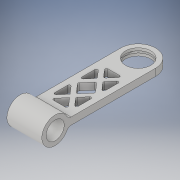
# Autodesk Inventor part: motor test flapper
Saved by Autodesk Inventor 2018.2 (Build 222227000, 227)
## iProperties
Created: 2018-03-04
Part Number: motor test flapper
Material: Generic
Document SubType Name: Modeling
Designer: torba
Density: 1 g/cm^3
Appearance: Default
Author: torba
Autodesk Inventor part; units mm, degrees
ref_plane "YZ Plane" through (0, 0, 0) normal (1, 0, 0) x (0, 1, 0)
ref_plane "XZ Plane" through (0, 0, 0) normal (0, 1, 0) x (-1, 0, 0)
sketch "Sketch1" plane through (0, 0, 0) normal (0, 1, 0) x (-1, 0, 0)
  line L0 (-12.25, 67.2283) -> (7.0949, 67.2283)
  arc A0 (-12.25, 3.0302) -> (12.25, 3.0302) centre (0, 3.0302) ccw
  line L1 (12.25, 3.0302) -> (12.25, 67.2283)
  line L2 (-12.25, 67.2283) -> (-12.25, 3.0302)
  line L3 (-12.25, 67.2283) -> (12.25, 67.2283)
  line L4 (12.25, 67.2283) -> (-12.25, 67.2283)
  circle A1 centre (0, 3.0302) radius 12.25
  point P0 (0, 0)
  dimension "d1" = 24.5
  dimension "d41" = 64.1981
  constraints: 10 end point, 2 equal length, 2 point on circle, 2 tangent, 1 centre point, 1 coincident, 1 horizontal, 1 horizontal alignment, 1 point on line, 4 other
  measures "d1" diameter of A0
  measures "d41" distance from line of point (0, 3.03) L3
extrude "Extrusion1" add sketch "Sketch1" along normal blind 5
sketch "Sketch3" plane through (12.25, 0, 67.2283) normal (1, 0, 0) x (0, 0, -1)
  line L0 (0, 0) -> (64.1981, 0) projected
  line L1 (64.1981, 0) -> (64.1981, 5) projected
  line L2 (0, 5) -> (64.1981, 5) projected
  line L3 (0, 0) -> (0, 5) projected
  line L4 (0, 2.5) -> (-6.35, 2.5)
  circle A0 centre (-6.35, 2.5) radius 6.35
  circle A1 centre (-6.35, 2.5) radius 9.35
  line L5 (0, 0) -> (0, 5) projected
  point P0 (67.2283, 0)
  dimension "d10" = 6.35
  dimension "d11" = 18.7
  constraints: 2 coincident, 2 end point, 1 centre point, 1 horizontal, 1 horizontal alignment, 1 midpoint, 2 other
  measures "d10" distance of L4.start L4.end
  measures "d11" diameter of A1
extrude "Extrusion2" add sketch "Sketch3" against normal up to surface (24.5 mm away) contours L3 L2 A1 L0 | L0 A1 L2 L3
fillet "Fillet1" radius 3.175 2 edges at (0, 5, 64.5687) (0, 0, 64.5687)
ref_plane "Work Plane1" through (0, 0, -9.2198) normal (0, 0, 1) x (1, 0, 0)
sketch "Sketch4" plane through (0, 0, -9.2198) normal (0, 0, 1) x (1, 0, 0)
  line L0 (12.25, 0) -> (-12.25, 0) projected
  line L1 (-12.25, 0) -> (-12.25, 5) projected
  line L2 (12.25, 5) -> (-12.25, 5) projected
  line L3 (12.25, 0) -> (12.25, 5) projected
  line L4 (0, 5) -> (0, 0)
  line L5 (9.125, 3.16) -> (-9.125, 3.16)
  line L6 (-9.125, 3.16) -> (-9.125, 1.84)
  line L7 (-9.125, 1.84) -> (9.125, 1.84)
  line L8 (9.125, 1.84) -> (9.125, 3.16)
  line L9 (9.125, 3.16) -> (-9.125, 1.84) construction
  line L10 (-9.125, 3.16) -> (9.125, 1.84) construction
  point P0 (0, 2.5)
  dimension "d15" = 18.25
  dimension "d16" = 1.32
  constraints: 14 end point, 4 midpoint, 2 parallel, 1 horizontal, 1 perpendicular, 1 vertical
  measures "d15" distance of L7.end L6.end
  measures "d16" distance of L6.end L5.end
extrude "Extrusion3" cut sketch "Sketch4" along normal blind 25.4 contours L7 L6 L5 L4 | L4 L5 L8 L7
sketch "Sketch5" plane through (0, 5, 0) normal (0, 1, 0) x (1, 0, 0)
  arc A0 (12.25, -3.0302) -> (-12.25, -3.0302) centre (0, -3.0302) ccw projected
  point P0 (0, 0)
hole "Hole1" at (0, 5, 3.0302) direction (0, -1, 0) diameter 17.78 depth 25.4 tip angle 118
sketch "Sketch6" plane through (0, 5, 0) normal (0, 1, 0) x (1, 0, 0)
  circle A0 centre (0, -3.0302) radius 8.89 projected
  line L0 (12.25, -62.4127) -> (-12.25, -62.4127) projected
  line L1 (12.25, -62.4127) -> (12.25, -3.0302) projected
  arc A1 (12.25, -3.0302) -> (-12.25, -3.0302) centre (0, -3.0302) ccw projected
  line L2 (-12.25, -3.0302) -> (-12.25, -62.4127) projected
  line L3 (-9.125, 5.1427) -> (-9.125, -16.1802) projected
  line L4 (9.125, -16.1802) -> (-9.125, -16.1802) projected
  line L5 (9.125, 5.1427) -> (9.125, -16.1802) projected
  line L6 (-8.25, -58.4127) -> (8.25, -58.4127)
  line L7 (8.25, -58.4127) -> (8.25, -20.1802)
  line L8 (8.25, -20.1802) -> (-8.25, -20.1802)
  line L9 (-8.25, -20.1802) -> (-8.25, -58.4127)
  line L10 (8.25, -58.4127) -> (-8.25, -39.2965)
  line L11 (8.25, -20.1802) -> (-8.25, -39.2965)
  line L12 (-8.25, -20.1802) -> (8.25, -39.2965)
  line L13 (-8.25, -58.4127) -> (8.25, -39.2965)
  point P0 (0, 0)
  dimension "d26" = 4
  dimension "d27" = 4
  dimension "d28" = 4
  dimension "d29" = 4
  constraints: 16 end point, 2 midpoint, 2 parallel, 1 horizontal, 1 perpendicular
  measures "d26" distance between parallel lines of L2 L9
  measures "d27" distance between parallel lines of L1 L7
  measures "d28" distance between parallel lines of L4 L8
  measures "d29" distance between parallel lines of L0 L6
extrude "Extrusion4" cut sketch "Sketch6" against normal blind 25.4 contours L13 L10 L6 | L9 L10 L13 | L10 L13 L7 | L11 L12 L13 L10 | L9 L12 L11 | L12 L11 L7 | L8 L11 L12
sketch "Sketch7" plane through (0, 5, 0) normal (0, 1, 0) x (1, 0, 0)
  line L0 (8.25, -20.1802) -> (8.25, -58.4127) projected
  line L1 (8.25, -58.4127) -> (-8.25, -58.4127) projected
  line L2 (-8.25, -58.4127) -> (-8.25, -20.1802) projected
  line L3 (-8.25, -20.1802) -> (8.25, -20.1802) projected
  circle A0 centre (0, -3.0302) radius 8.89 projected
  line L4 (12.25, -62.4127) -> (-12.25, -62.4127) projected
  line L5 (12.25, -62.4127) -> (12.25, -3.0302) projected
  arc A1 (12.25, -3.0302) -> (-12.25, -3.0302) centre (0, -3.0302) ccw projected
  line L6 (-12.25, -3.0302) -> (-12.25, -62.4127) projected
  line L7 (8.25, -58.4127) -> (-8.25, -58.4127) projected
  line L8 (-8.25, -58.4127) -> (8.25, -39.2965) construction
  line L9 (8.25, -20.1802) -> (8.25, -58.4127) projected
  line L10 (-8.25, -20.1802) -> (8.25, -39.2965) construction
  line L11 (8.25, -20.1802) -> (-8.25, -39.2965) construction
  line L12 (-8.25, -58.4127) -> (-8.25, -20.1802) projected
  line L13 (8.25, -58.4127) -> (-8.25, -39.2965) construction
  line L14 (-8.25, -58.4127) -> (8.25, -39.2965) construction
  line L15 (-6.1344, -58.2573) -> (8.4054, -41.4121)
  line L16 (6.1344, -39.4519) -> (-8.4054, -56.2971)
  arc A2 (-8.4054, -56.2971) -> (-6.1344, -58.2573) centre (-7.2699, -57.2772) ccw
  arc A3 (8.4054, -41.4121) -> (6.1344, -39.4519) centre (7.2699, -40.432) ccw
  line L17 (8.25, -58.4127) -> (-8.25, -39.2965) construction
  line L18 (8.4054, -56.2971) -> (-6.1344, -39.4519)
  line L19 (-8.4054, -41.4121) -> (6.1344, -58.2573)
  arc A4 (6.1344, -58.2573) -> (8.4054, -56.2971) centre (7.2699, -57.2772) ccw
  arc A5 (-6.1344, -39.4519) -> (-8.4054, -41.4121) centre (-7.2699, -40.432) ccw
  line L20 (8.25, -20.1802) -> (-8.25, -39.2965) construction
  line L21 (6.1344, -20.3356) -> (-8.4054, -37.1809)
  line L22 (-6.1344, -39.1411) -> (8.4054, -22.2959)
  arc A6 (8.4054, -22.2959) -> (6.1344, -20.3356) centre (7.2699, -21.3157) ccw
  arc A7 (-8.4054, -37.1809) -> (-6.1344, -39.1411) centre (-7.2699, -38.161) ccw
  line L23 (8.25, -20.1802) -> (-8.25, -20.1802) projected
  line L24 (-8.25, -20.1802) -> (8.25, -39.2965) construction
  line L25 (-8.4054, -22.2959) -> (6.1344, -39.1411)
  line L26 (8.4054, -37.1809) -> (-6.1344, -20.3356)
  arc A8 (-6.1344, -20.3356) -> (-8.4054, -22.2959) centre (-7.2699, -21.3157) ccw
  arc A9 (6.1344, -39.1411) -> (8.4054, -37.1809) centre (7.2699, -38.161) ccw
  point P0 (0, 0)
  point P1 (0, -48.8546)
  point P2 (0, -48.8546)
  point P3 (0, -29.7384)
  point P4 (0, -29.7384)
  dimension "d32" = 3
  dimension "d33" = 3
  dimension "d34" = 3
  dimension "d35" = 3
  constraints: 40 end point, 25 point on circle, 16 tangent, 10 point on line, 8 centre point, 7 midpoint, 7 parallel, 1 collinear
  measures "d32" diameter of A3
  measures "d33" diameter of A5
  measures "d34" diameter of A7
  measures "d35" diameter of A9
extrude "Extrusion5" add sketch "Sketch7" against normal up to surface (5 mm away) contours A6 L22 L0 | L0 L22 L26 L21 A6 L3 | L3 A6 | L26 A9 L0 | L0 A3 A9 L25 L22 L26 | L22 L25 L21 L26 | A8 L26 L21 L25 L2 L3 | L3 A8 | A3 L15 L0 | A9 A3 | L0 L15 L18 L16 A3 A9 | L22 A7 A5 L2 L21 L25 | L2 L25 A8 | L18 A4 L0 | L0 L1 A4 L19 L15 L18 | L15 L19 L16 L18 | A7 A5 | A5 L18 L16 L19 L2 A7 | L2 A7 L21 | A4 L1 | L15 A2 L1 L2 L16 L19 | L2 L19 A5 | A2 L1 | L2 A2 L16
fillet "Fillet2" radius 1 20 edges at (1.9815, 2.5, 48.8546) (-6.2898, 2.5, 58.4127) (-6.2898, 2.5, 39.2965) (1.9815, 2.5, 29.7384) (0, 2.5, 32.034) (8.25, 2.5, 22.4759) (-6.2898, 2.5, 20.1802) (-8.25, 2.5, 22.4759) (-8.25, 2.5, 41.5922) (-8.25, 2.5, 56.1171) (0, 2.5, 46.5589) (8.25, 2.5, 37.0008) (6.2898, 2.5, 39.2965) (8.25, 2.5, 41.5922) (8.25, 2.5, 56.1171) (6.2898, 2.5, 58.4127) (-8.25, 2.5, 37.0008) (6.2898, 2.5, 20.1802) (-1.9815, 2.5, 29.7384) (0, 2.5, 27.4427)
body "Solid1"
